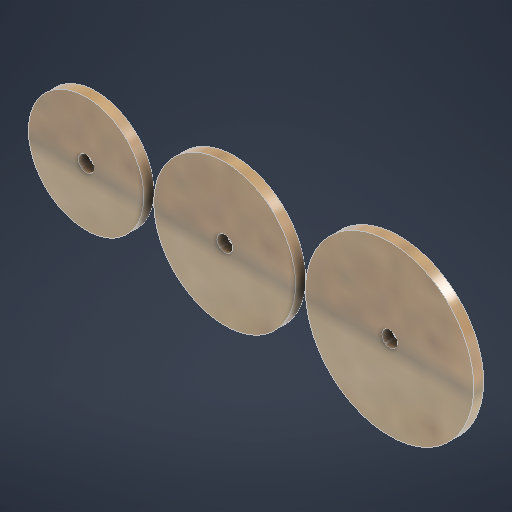
# Autodesk Inventor part: wheels
Saved by Autodesk Inventor 2025.3 (Build 293356030, 356C)
## iProperties
Created: 2025-09-04
Part Number: wheels
Material: 木材 (楓木)
Document SubType Name: Modeling
Designer: 陳泓任
Density: 0.67 g/cm^3
Appearance: 天然楓木 - 深色亮面處理
Author: 陳泓任
Autodesk Inventor part; units mm, degrees
ref_plane "YZ Plane" through (0, 0, 0) normal (1, 0, 0) x (0, 1, 0)
ref_plane "XZ Plane" through (0, 0, 0) normal (0, 1, 0) x (-1, 0, 0)
ref_plane "XY Plane" through (0, 0, 0) normal (0, 0, 1) x (1, 0, 0)
sketch "草圖1" plane through (0, 0, 0) normal (0, 0, 1) x (1, 0, 0)
  circle A0 centre (0, 0) radius 17.5
  circle A1 centre (42, 0) radius 21.5
  circle A2 centre (92, 0) radius 25.5
  circle A3 centre (0, 0) radius 2.34
  circle A4 centre (42, 0) radius 2.34
  circle A5 centre (92, 0) radius 2.34
  line L0 (0, 0) -> (92, 0)
  dimension "d0" = 35
  dimension "d1" = 43
  dimension "d2" = 51
  dimension "d3" = 4.68
  dimension "d4" = 42
  dimension "d5" = 50
  constraints: 6 centre point, 4 coincident, 2 end point, 2 equal radius, 1 horizontal, 1 point on line
  measures "d0" diameter of A0
  measures "d1" diameter of A1
  measures "d2" diameter of A2
  measures "d3" diameter of A3
  measures "d4" distance of A1.centre A0.centre
  measures "d5" distance of A1.centre A2.centre
extrude "擠出1" add sketch "草圖1" along normal blind 3 contours A0
extrude "擠出2" add sketch "草圖1" along normal blind 3 separate body contours L0 A4 A1 | A1 L0 A4
extrude "擠出3" add sketch "草圖1" along normal blind 3 separate body contours A2
